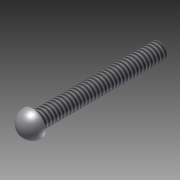
# Autodesk Inventor part: screw
Saved by Autodesk Inventor 2011 (Build 150239000, 239)
## iProperties
Created: 2013-01-27
Part Number: screw
Document SubType Name: Modeling
Designer: Danny
Density: 1 g/cm^3
Author: Danny
Autodesk Inventor part; units mm, degrees
ref_plane "YZ Plane" through (0, 0, 0) normal (1, 0, 0) x (0, 1, 0)
ref_plane "XZ Plane" through (0, 0, 0) normal (0, 1, 0) x (-1, 0, 0)
ref_plane "XY Plane" through (0, 0, 0) normal (0, 0, 1) x (1, 0, 0)
sketch "Sketch1" plane through (0, 0, 0) normal (0, 0, 1) x (1, 0, 0)
  circle A0 centre (0, 0) radius 2.3813
  dimension "d0" = 4.7625
  constraints: 1 centre point, 1 coincident
  measures "d0" diameter of A0
extrude "Extrusion1" add sketch "Sketch1" along normal blind 38.1
sketch "Sketch2" plane through (0, 0, 38.1) normal (0, 0, 1) x (1, 0, 0)
  circle A0 centre (0, 0) radius 2.3813 projected
  arc A1 (-3.81, 0) -> (3.81, 0) centre (0, 0) ccw
  line L0 (-3.81, 0) -> (3.81, 0)
  arc A2 (3.81, 0) -> (-3.81, 0) centre (0, 0) ccw
  dimension "d3" = 7.62
  constraints: 4 point on circle, 2 centre point, 2 end point, 1 coincident, 1 horizontal
  measures "d3" diameter of A1
revolve "Revolution1" add sketch "Sketch2" angle 180 about axis through (-3.81, 0, 38.1) along (1, 0, 0) picked at (0.5941, 0.5264) contours L0 A0 | A0 L0 A2
thread "Thread1" size "10-24 UNC" class "2A" standard "ANSI Unified Screw Threads" full length
chamfer "Chamfer1" distance 0.381 angle 45 1 edges at (-2.3813, 0, 0)
body "Solid1"
